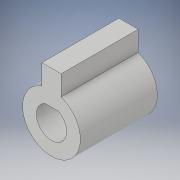
# Autodesk Inventor part: Seeder Motor Gear key
Saved by Autodesk Inventor 2017 (Build 210142000, 142)
## iProperties
Created: 2017-05-24
Part Number: Seeder Motor Gear key
Material: Generic
Document SubType Name: Modeling
Designer: Jon
Density: 1 g/cm^3
Appearance: Default
Author: Jon
Autodesk Inventor part; units mm, degrees
ref_plane "YZ Plane" through (0, 0, 0) normal (1, 0, 0) x (0, 1, 0)
ref_plane "XZ Plane" through (0, 0, 0) normal (0, 1, 0) x (-1, 0, 0)
ref_plane "XY Plane" through (0, 0, 0) normal (0, 0, 1) x (1, 0, 0)
sketch "Sketch1" plane through (0, 0, 0) normal (0, 0, 1) x (1, 0, 0)
  arc A0 (-3.175, 8.9803) -> (3.175, 8.9803) centre (0, 0) ccw
  line L0 (-3.175, 15.621) -> (3.175, 15.621)
  line L1 (3.175, 15.621) -> (3.175, 8.9803)
  line L2 (-3.175, 8.9803) -> (-3.175, 15.621)
  dimension "d0" = 19.05
  dimension "d1" = 6.35
  constraints: 6 end point, 2 point on circle, 1 centre point, 1 coincident, 1 horizontal, 1 parallel, 1 perpendicular
  measures "d0" diameter of A0
  measures "d1" distance of L0.start L0.end
extrude "Extrusion1" add sketch "Sketch1" along normal blind 25.4
sketch "Sketch2" plane through (0, 0, 25.4) normal (0, 0, 1) x (1, 0, 0)
  arc A0 (-2.1794, 4.5) -> (2.1794, 4.5) centre (0, 0) ccw
  line L0 (-2.1794, 4.5) -> (2.1794, 4.5)
  dimension "d7" = 10
  dimension "d8" = 9.5
  constraints: 2 end point, 2 point on circle, 1 centre point, 1 coincident, 1 horizontal
  measures "d7" diameter of A0
extrude "Extrusion2" cut sketch "Sketch2" against normal blind 25.4
body "Solid1"
